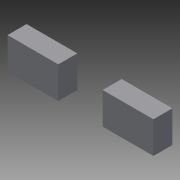
# Autodesk Inventor part: GapBumper
Saved by Autodesk Inventor 2013 (Build 170138000, 138)
## iProperties
Created: 2014-01-11
Part Number: GapBumper
Material: Generic
Document SubType Name: Modeling
Designer: 215152
Density: 1 g/cm^3
Author: 215152
Autodesk Inventor part; units mm, degrees
ref_plane "YZ Plane" through (0, 0, 0) normal (1, 0, 0) x (0, 1, 0)
ref_plane "XZ Plane" through (0, 0, 0) normal (0, 1, 0) x (-1, 0, 0)
ref_plane "XY Plane" through (0, 0, 0) normal (0, 0, 1) x (1, 0, 0)
sketch "Sketch1" plane through (0, 0, 0) normal (0, 0, 1) x (1, 0, 0)
  line L0 (0, 0) -> (203.2, 0)
  line L1 (203.2, 0) -> (203.2, 127)
  line L2 (203.2, 127) -> (0, 127)
  line L3 (0, 127) -> (0, 0)
  line L4 (0, 127) -> (584.2, 127)
  line L5 (584.2, 127) -> (584.2, 0)
  line L6 (584.2, 0) -> (0, 0)
  line L7 (0, 0) -> (0, 127)
  line L8 (584.2, 127) -> (381, 127)
  line L9 (381, 127) -> (381, 0)
  line L10 (381, 0) -> (584.2, 0)
  line L11 (584.2, 0) -> (584.2, 127)
  dimension "d0" = 203.2
  dimension "d1" = 127
  dimension "d2" = 584.2
  dimension "d3" = 127
  dimension "d4" = 203.2
  dimension "d5" = 127
  constraints: 24 end point, 6 parallel, 3 horizontal, 3 perpendicular
  measures "d0" distance of L2.end L1.end
  measures "d1" distance of L1.end L0.end
  measures "d2" distance of L5.end L6.end
  measures "d3" distance of L4.end L5.end
  measures "d4" distance of L10.end L9.end
  measures "d5" distance of L9.end L8.end
extrude "Extrusion1" add sketch "Sketch1" along normal blind 76.2 contours L3 L2 L1 L0 | L9 L4 L5 L6
body "Solid1"
